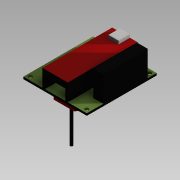
# Autodesk Inventor part: CarteElectronique
Saved by Autodesk Inventor 2014 (Build 180170000, 170)
## iProperties
Created: 2013-11-13
Part Number: CarteElectronique
Material: Générique
Document SubType Name: Modeling
Designer: Grégoire
Density: 1 g/cm^3
Appearance: Par défaut
Author: Grégoire
Autodesk Inventor part; units mm, degrees
ref_plane "YZ Plane" through (0, 0, 0) normal (1, 0, 0) x (0, 1, 0)
ref_plane "XZ Plane" through (0, 0, 0) normal (0, 1, 0) x (-1, 0, 0)
ref_plane "XY Plane" through (0, 0, 0) normal (0, 0, 1) x (1, 0, 0)
sketch "Esquisse1" plane through (0, 0, 0) normal (0, 0, 1) x (1, 0, 0)
  line L0 (0, 0) -> (50, 0)
  line L1 (50, 0) -> (50, 55)
  line L2 (50, 55) -> (0, 55)
  line L3 (0, 55) -> (0, 0)
  dimension "d0" = 50
  dimension "d1" = 55
  constraints: 8 end point, 2 parallel, 1 horizontal, 1 perpendicular
  measures "d0" distance of L0.start L0.end
  measures "d1" distance of L2.end L0.start
extrude "Extrusion1" add sketch "Esquisse1" along normal blind 1.7
sketch "Esquisse2" plane through (0, 0, 1.7) normal (0, 0, 1) x (1, 0, 0)
  line L0 (0, 0) -> (50, 0) construction
  line L1 (50, 0) -> (50, 55) construction
  line L2 (50, 55) -> (0, 55) construction
  line L3 (0, 55) -> (0, 0) construction
  line L4 (25, 55) -> (25, 0) construction
  line L5 (0, 27.5) -> (50, 27.5) construction
  circle A0 centre (2.8, 52.2) radius 1.5
  line L6 (2.8, 52.2) -> (2.8, 55) construction
  line L7 (2.8, 52.2) -> (0, 52.2) construction
  circle A1 centre (47.2, 52.2) radius 1.5
  circle A2 centre (2.8, 2.8) radius 1.5
  circle A3 centre (47.2, 2.8) radius 1.5
  dimension "d4" = 2.8
  dimension "d5" = 3
  constraints: 8 end point, 4 centre point, 4 midpoint, 3 perpendicular, 3 symmetric about line, 2 point on line, 3 other
  measures "d4" distance of L6.start L6.end
  measures "d5" diameter of A0
extrude "Extrusion2" cut sketch "Esquisse2" against normal blind 1.7
sketch "Esquisse3" plane through (0, 0, 1.7) normal (0, 0, 1) x (1, 0, 0)
  line L0 (50, 0) -> (50, 55) construction
  line L1 (0, 55) -> (0, 0) construction
  line L2 (15, 55) -> (35, 55)
  line L3 (35, 55) -> (35, 0)
  line L4 (35, 0) -> (15, 0)
  line L5 (15, 0) -> (15, 55)
  line L6 (15, 27.5) -> (0, 27.5) construction
  line L7 (35, 27.5) -> (50, 27.5) construction
  dimension "d8" = 20
  dimension "d9" = 55
  constraints: 12 end point, 4 midpoint, 2 parallel, 2 perpendicular, 1 collinear, 1 horizontal
  measures "d8" distance of L2.start L2.end
  measures "d9" distance of L2.end L3.end
extrude "Extrusion3" add sketch "Esquisse3" along normal blind 8.5
sketch "Esquisse4" plane through (0, 0, 0) normal (0, -1, 0) x (1, 0, 0)
  line L0 (0, 0) -> (50, 0) projected
  line L1 (35, 1.7) -> (50, 1.7) projected
  line L2 (35, 1.7) -> (35, 10.2) projected
  line L3 (15, 10.2) -> (35, 10.2) projected
  line L4 (15, 1.7) -> (15, 10.2) projected
  line L5 (17, 10.2) -> (33, 10.2)
  line L6 (33, 10.2) -> (33, 1.7)
  line L7 (33, 1.7) -> (17, 1.7)
  line L8 (17, 1.7) -> (17, 10.2)
  line L9 (25, 1.7) -> (25, 0) construction
  line L10 (39.3041, 1.7) -> (39.3041, 0) construction
  dimension "d12" = 2
  dimension "d13" = 2
  constraints: 12 end point, 3 parallel, 3 point on line, 2 midpoint, 2 perpendicular, 1 horizontal
  measures "d12" distance between parallel lines of L4 L8
  measures "d13" distance between parallel lines of L2 L6
extrude "Extrusion4" cut sketch "Esquisse4" against normal through all
sketch "Esquisse5" plane through (0, 0, 10.2) normal (0, 0, 1) x (1, 0, 0)
  line L0 (33, 55) -> (33, 0) construction
  line L1 (35, 55) -> (33, 55) construction
  line L2 (35, 0) -> (35, 55) construction
  line L3 (33, 0) -> (35, 0) construction
  line L4 (15, 55) -> (35, 55)
  line L5 (35, 55) -> (35, 0)
  line L6 (35, 0) -> (15, 0)
  line L7 (15, 0) -> (15, 55)
  point P0 (0, 0)
  constraints: 8 end point, 2 parallel, 1 horizontal, 1 perpendicular
extrude "Extrusion5" add sketch "Esquisse5" along normal blind 5
sketch "Esquisse6" plane through (0, 0, 15.2) normal (0, 0, 1) x (1, 0, 0)
  line L0 (35, 55) -> (15, 55) construction
  line L1 (15, 55) -> (15, 0) construction
  line L2 (35, 0) -> (35, 55) construction
  line L3 (21, 55) -> (29, 55)
  line L4 (29, 55) -> (29, 46)
  line L5 (29, 46) -> (21, 46)
  line L6 (21, 46) -> (21, 55)
  line L7 (21, 50.5) -> (15, 50.5) construction
  line L8 (29, 50.5) -> (35, 50.5) construction
  point P0 (0, 0)
  dimension "d18" = 8
  dimension "d19" = 9
  constraints: 12 end point, 3 equal length, 3 point on line, 2 midpoint, 2 perpendicular, 1 collinear, 1 horizontal
  measures "d18" distance of L4.end L5.end
  measures "d19" distance of L5.end L3.start
extrude "Extrusion6" add sketch "Esquisse6" along normal blind 2.5
sketch "Esquisse7" plane through (0, 0, 0) normal (0, 0, -1) x (-1, 0, 0)
  line L0 (0, 0) -> (-50, 0) construction
  line L1 (0, 55) -> (0, 0) construction
  line L2 (-50, 0) -> (-50, 55) construction
  line L3 (-37, 40) -> (-13, 40)
  line L4 (-13, 40) -> (-13, 12.7126)
  line L5 (-17, 7) -> (-33, 7)
  line L6 (-37, 12.7126) -> (-37, 40)
  line L7 (-37, 23.5) -> (-50, 23.5) construction
  line L8 (-13, 23.5) -> (0, 23.5) construction
  line L9 (-37, 12.7126) -> (-33, 7)
  line L10 (-17, 7) -> (-13, 12.7126)
  dimension "d23" = 7
  dimension "d24" = 24
  dimension "d28" = 145
  dimension "d29" = 145
  dimension "d30" = 33
  dimension "d31" = 4
  constraints: 16 end point, 4 point on line, 3 perpendicular, 2 equal length, 2 parallel, 1 horizontal
  measures "d23" distance between parallel lines of L0 L5
  measures "d24" distance of L3.start L3.end
  measures "d28" angle of L6 L9
  measures "d29" angle of L4 L10
  measures "d30" distance between parallel lines of L5 L3
  measures "d31" horizontal distance of L6.start L5.end
extrude "Extrusion7" add sketch "Esquisse7" along normal blind 9
sketch "Esquisse8" plane through (0, 0, -9) normal (0, 0, -1) x (-1, 0, 0)
  line L0 (-17, 7) -> (-13, 12.7126) construction
  line L1 (-13, 12.7126) -> (-13, 40) construction
  circle A0 centre (-25.1584, 12.7126) radius 1
  line L2 (-13, 12.7126) -> (-37, 12.7126) construction
  line L3 (-33, 7) -> (-25.1584, 12.7126) construction
  line L4 (-25.1584, 12.7126) -> (-17, 7) construction
  point P0 (0, 0)
  dimension "d32" = 2
  constraints: 6 end point, 2 perpendicular, 1 centre point, 1 point on line
  measures "d32" diameter of A0
extrude "Extrusion8" add sketch "Esquisse8" along normal blind 30
sketch "Esquisse9" plane through (0, 0, 1.7) normal (0, 0, 1) x (1, 0, 0)
  line L0 (50, 0) -> (50, 55) construction
  line L1 (50, 55) -> (35, 55) construction
  line L2 (50, 48) -> (42, 48)
  line L3 (42, 48) -> (42, 13)
  line L4 (42, 13) -> (50, 13)
  line L5 (50, 13) -> (50, 48)
  line L6 (42, 48) -> (42, 55) construction
  point P0 (0, 0)
  dimension "d35" = 0
  dimension "d36" = 8
  dimension "d37" = 35
  dimension "d38" = 7
  constraints: 10 end point, 2 parallel, 2 perpendicular, 1 horizontal, 1 point on line
  measures "d35" distance between parallel lines of L0 L5
  measures "d36" distance of L3.end L4.end
  measures "d37" distance of L2.end L3.end
  measures "d38" distance of L2.end L6.end
extrude "Extrusion9" add sketch "Esquisse9" along normal blind 20
equation "\"d13\" = d12"
equation "\"d29\" = d28"
